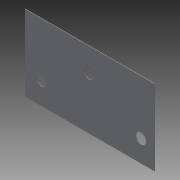
# Autodesk Inventor part: Panel
Saved by Autodesk Inventor 2015 (Build 190159000, 159)
## iProperties
Created: 2015-04-03
Part Number: Panel
Material: Generic
Document SubType Name: Modeling
Designer: Matthew
Density: 1 g/cm^3
Appearance: Default
Author: Matthew
Autodesk Inventor part; units mm, degrees
ref_plane "YZ Plane" through (0, 0, 0) normal (1, 0, 0) x (0, 1, 0)
ref_plane "XZ Plane" through (0, 0, 0) normal (0, 1, 0) x (-1, 0, 0)
ref_plane "XY Plane" through (0, 0, 0) normal (0, 0, 1) x (1, 0, 0)
sketch "Sketch1" plane through (0, 0, 0) normal (0, 0, 1) x (1, 0, 0)
  line L0 (-363.5144, 243.2472) -> (135.0368, 243.2472)
  line L1 (135.0368, 243.2472) -> (135.0368, -47.8114)
  line L2 (135.0368, -47.8114) -> (-363.5144, -47.8114)
  line L3 (-363.5144, -47.8114) -> (-363.5144, 243.2472)
  point P0 (0, 0)
  dimension "d0" = 498.5512
  dimension "d1" = 291.0586
  constraints: 8 end point, 2 parallel, 1 horizontal, 1 perpendicular
  measures "d0" distance of L0.start L0.end
  measures "d1" distance of L2.end L0.start
extrude "Extrusion1" add sketch "Sketch1" along normal blind 2.0066
sketch "Sketch2" plane through (0, 0, 2.0066) normal (0, 0, 1) x (1, 0, 0)
  circle A0 centre (82.6198, 35.0228) radius 19.7358
  circle A1 centre (66.3698, 18.7728) radius 1.25
  line L0 (385.8263, -153.0596) -> (385.8263, 254.4224)
  line L1 (-77.3983, -47.0364) -> (620.5734, -47.0364)
  circle A2 centre (66.3698, 51.2728) radius 1.25
  circle A3 centre (98.8698, 18.7728) radius 1.25
  circle A4 centre (98.8698, 51.2728) radius 1.25
  point P0 (385.8263, -47.0364)
  dimension "d4" = 39.4716
  dimension "d5" = 2.5
  dimension "d11" = 32.5
  dimension "d14" = 32.5
  dimension "d17" = 16.25
  dimension "d18" = 16.25
  constraints: 5 centre point, 4 end point, 1 horizontal, 1 vertical, 6 other
  measures "d4" diameter of A0
  measures "d5" diameter of A1
  measures "d11" distance of A1.centre A2.centre
  measures "d14" distance of A1.centre A3.centre
  measures "d17" horizontal distance of A0.centre A2.centre
  measures "d18" horizontal distance of A1.centre A0.centre
extrude "Joystick 1" cut sketch "Sketch2" against normal blind 2.0066
sketch "Sketch3" plane through (1.6331, 0.1353, 2.0066) normal (0, 0, 1) x (1, 0, 0)
  circle A0 centre (-301.0067, 37.2418) radius 19.7358
  circle A1 centre (-317.2567, 20.9918) radius 1.25
  line L0 (0, -106.0232) -> (0, 301.4589)
  line L1 (-463.2246, 0) -> (234.7471, 0)
  circle A2 centre (-317.2567, 53.4918) radius 1.25
  circle A3 centre (-284.7567, 20.9918) radius 1.25
  circle A4 centre (-284.7567, 53.4918) radius 1.25
  point P0 (0, 0)
  dimension "d30" = 39.4716
  dimension "d28" = 2.5
  dimension "d22" = 32.5
  dimension "d21" = 32.5
  dimension "d27" = 16.25
  dimension "d29" = 16.25
  constraints: 5 centre point, 4 end point, 1 horizontal, 1 vertical, 6 other
  measures "d30" diameter of A0
  measures "d28" diameter of A1
  measures "d22" distance of A1.centre A2.centre
  measures "d21" distance of A1.centre A3.centre
  measures "d27" horizontal distance of A0.centre A2.centre
  measures "d29" horizontal distance of A1.centre A0.centre
extrude "Joystick 2" cut sketch "Sketch3" against normal blind 2.0066
sketch "Sketch4" plane through (0, 0, 2.0066) normal (0, 0, 1) x (1, 0, 0)
  circle A0 centre (-117.2987, 153.872) radius 21.5
  circle A1 centre (-117.2987, 179.272) radius 1.75
  circle A2 centre (-139.2957, 141.172) radius 1.75
  circle A3 centre (-95.3016, 141.172) radius 1.75
  point P0 (0, 0)
  dimension "d34" = 43
  dimension "d35" = 25.4
  dimension "d36" = 3.5
  dimension "d39" = 360
  constraints: 4 centre point, 1 vertical alignment, 7 other
  measures "d34" diameter of A0
  measures "d35" distance of A0.centre A1.centre
  measures "d36" diameter of A1
extrude "Throttle Encoder" cut sketch "Sketch4" against normal blind 2.0066
body "Solid1"
